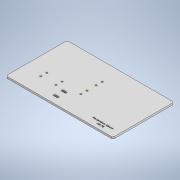
# Autodesk Inventor part: base
Saved by Autodesk Inventor 2022 (Build 260153000, 153)
## iProperties
Created: 2022-02-04
Part Number: base
Material: Generic
Document SubType Name: Modeling
Designer: Home
Density: 1 g/cm^3
Appearance: Default
Author: Home
Autodesk Inventor part; units mm, degrees
ref_plane "YZ Plane" through (0, 0, 0) normal (1, 0, 0) x (0, 1, 0)
ref_plane "XZ Plane" through (0, 0, 0) normal (0, 1, 0) x (-1, 0, 0)
ref_plane "XY Plane" through (0, 0, 0) normal (0, 0, 1) x (1, 0, 0)
sketch "Sketch1" plane through (0, 0, 0) normal (0, 1, 0) x (-1, 0, 0)
  line L0 (175, 100) -> (-175, 100)
  line L1 (-175, 100) -> (-175, -100)
  line L2 (-175, -100) -> (175, -100)
  line L3 (175, -100) -> (175, 100)
  line L4 (175, 100) -> (-175, -100) construction
  line L5 (-175, 100) -> (175, -100) construction
  point P0 (0, 0)
  dimension "d0" = 350
  dimension "d1" = 200
  constraints: 12 end point, 2 midpoint, 2 parallel, 1 horizontal, 1 perpendicular
  measures "d0" distance of L2.end L1.end
  measures "d1" distance of L1.end L0.end
extrude "Extrusion1" add sketch "Sketch1" along normal blind 6
fillet "Fillet1" radius 5 4 edges at (175, 3, 100) (175, 3, -100) (-175, 3, 100) (-175, 3, -100)
sketch "Sketch2" plane through (0, 6, 0) normal (0, 1, 0) x (1, 0, 0)
  line L0 (70.7569, -69.3202) -> (168.4517, -69.3202) construction
  line L1 (168.4517, -69.3202) -> (168.4517, -91.5888) construction
  line L2 (168.4517, -91.5888) -> (70.7569, -91.5888) construction
  line L3 (70.7569, -91.5888) -> (70.7569, -69.3202) construction
  point P0 (0, 0)
  constraints: 2 other
sketch "Sketch3" plane through (0, 6, 0) normal (0, 1, 0) x (1, 0, 0)
  line L0 (-175, 95) -> (-175, -95) projected
  line L1 (-170, -100) -> (170, -100) projected
  line L2 (170, 100) -> (-170, 100) projected
  line L3 (-42.5, -47) -> (-27.5, -47)
  line L4 (-27.5, -47) -> (-27.5, -53)
  line L5 (-27.5, -53) -> (-42.5, -53)
  line L6 (-42.5, -53) -> (-42.5, -47)
  line L7 (-42.5, -47) -> (-27.5, -53) construction
  line L8 (-27.5, -47) -> (-42.5, -53) construction
  line L9 (0, 140) -> (0, -140) projected
  line L10 (245, 0) -> (-245, 0) projected
  line L11 (-42.5, -73) -> (-27.5, -73)
  line L12 (-27.5, -73) -> (-27.5, -79)
  line L13 (-27.5, -79) -> (-42.5, -79)
  line L14 (-42.5, -79) -> (-42.5, -73)
  line L15 (-42.5, -73) -> (-27.5, -79) construction
  line L16 (-27.5, -73) -> (-42.5, -79) construction
  point P0 (0, 0)
  point P1 (0, 20)
  point P2 (0, 40)
  point P3 (0, -10)
  point P4 (0, -30)
  point P5 (-116.5, -45)
  point P6 (-116.5, -25)
  point P7 (-66.5, -25)
  point P8 (-66.5, -45)
  point P9 (-35, -50)
  point P10 (-35, -76)
  dimension "d7" = 20
  dimension "d8" = 20
  dimension "d18" = 20
  dimension "d19" = 20
  dimension "d20" = 50
  dimension "d21" = 58.5
  dimension "d22" = 55
  dimension "d23" = 60
  dimension "d24" = 30
  dimension "d25" = 15
  dimension "d26" = 6
  dimension "d27" = 35
  dimension "d30" = 50
  dimension "d31" = 15
  dimension "d32" = 6
  dimension "d33" = 35
  dimension "d34" = 20
  constraints: 24 end point, 5 vertical alignment, 4 midpoint, 4 parallel, 2 horizontal, 2 horizontal alignment, 2 perpendicular
  measures "d7" distance of point (0, 20) point (0, 40)
  measures "d8" distance of point (0, -30) point (0, -10)
  measures "d18" distance of point (-116.5, -45) point (-116.5, -25)
  measures "d19" distance of point (-66.5, -25) point (-66.5, -45)
  measures "d20" distance of point (-116.5, -45) point (-66.5, -45)
  measures "d21" distance from line of L0 point (-116.5, -25)
  measures "d22" distance from line of point (-116.5, -45) L1
  measures "d23" distance from line of L2 point (0, 40)
  measures "d24" distance of point (0, -10) point (0, 20)
  measures "d25" distance of L4.end L5.end
  measures "d26" distance of L3.end L4.end
  measures "d27" distance from line of L9 point (-35, -50)
  measures "d30" distance from line of L10 point (-35, -50)
  measures "d31" distance of L12.end L14.start
  measures "d32" distance of L11.end L12.end
  measures "d33" distance from line of L9 point (-35, -76)
  measures "d34" distance between parallel lines of L11 L5
hole "Hole1" at (0, 6, -40) at (0, 6, 30) at (0, 6, 10) at (0, 6, -20) at (-116.5, 6, 45) at (-116.5, 6, 25) at (-66.5, 6, 25) at (-66.5, 6, 45) direction (0, -1, 0) diameter 5.4 end through all
extrude "Extrusion2" cut sketch "Sketch3" against normal through all
equation "\"d8\" = d7"
equation "\"d19\" = d18"
equation "\"d33\" = d27"
body "Solid1"
